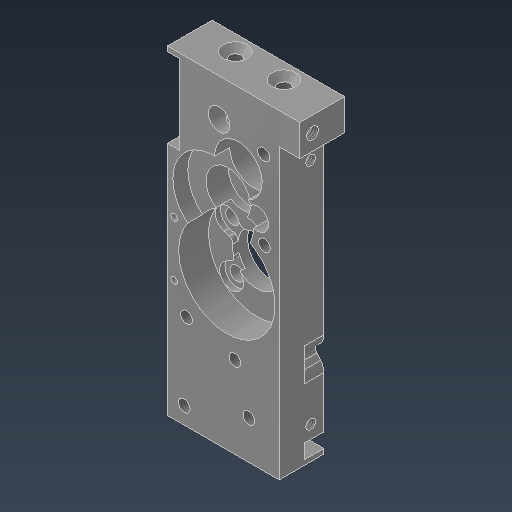
# Autodesk Inventor part: RightGearbox
Saved by Autodesk Inventor 2027.1 (Build 311270010, 270A)
## iProperties
Created: 2026-04-14
Part Number: RightGearbox
Material: Steel
Document SubType Name: Sheet Metal
Designer: szymo
Density: 7.85 g/cm^3
Appearance: Nylon 6(1)
Mass: 69.272 g
Surface Area: 68.2976 cm^2
Volume: 8.82446 cm^3
Sheet Metal Rule: Default
Author: szymo
Autodesk Inventor part; units mm, degrees
(part 1 of 2)
ref_plane "YZ Plane" through (0, 0, 0) normal (1, 0, 0) x (0, 1, 0)
sketch "Sketch1" plane through (0, 0, 0) normal (0, 0, 1) x (1, 0, 0)
  circle A0 centre (14.75, -14.75) radius 4.929289
  circle A1 centre (14.75, -14.75) radius 14.75 construction
  circle A2 centre (14.7, -55.637072) radius 4.955917
  circle A3 centre (14.7, -55.637072) radius 15.294083 construction
  line L0 (23.2, 0) -> (0, 0)
  line L1 (0, 0) -> (0, -66.431155)
  line L2 (0, -66.431155) -> (23.2, -66.431155)
  line L3 (23.2, -66.431155) -> (23.2, 0)
  circle A4 centre (12.35, -35.568116) radius 5
  line L4 (24.683483, -55.062556) -> (28.658141, -52.767786)
  arc A5 (28.658141, -52.767786) -> (24.908656, -45.694948) centre (14.7, -55.637072) ccw
  line L5 (24.908656, -45.694948) -> (21.057709, -47.918294)
  arc A6 (24.683483, -55.062556) -> (21.057709, -47.918294) centre (14.7, -55.637072) ccw construction
  arc A7 (25.213326, -45.342329) -> (3.718756, -65.431155) centre (14.7, -55.637072) ccw
  line L6 (25.213326, -45.342329) -> (3.904013, -59.159587)
  line L7 (6.945596, -62.431155) -> (3.718756, -65.431155)
  line L8 (24.683483, -55.062556) -> (23.2, -55.062556)
  line L9 (24.908656, -45.694948) -> (23.2, -45.694948)
  line L10 (6.945596, -62.431155) -> (3.904013, -59.159587)
  line L11 (24.683483, -55.062556) -> (21.057709, -47.918294)
  line L12 (6.945596, -62.431155) -> (23.2, -62.431155)
  circle A8 centre (9.53986, -23.285481) radius 4.2 construction
  circle A9 centre (9.53986, -23.285481) radius 8 construction
  circle A10 centre (12.35, -35.568116) radius 9.6 construction
  circle A11 centre (12.35, -35.568116) radius 10
  circle A12 centre (9.53986, -23.285481) radius 4.6
  circle A13 centre (9.53986, -23.285481) radius 8.4
  arc A14 (5.920333, -57.852177) -> (6.945596, -62.431155) centre (14.911835, -58.243191) ccw construction
  line L13 (2.5, -1) -> (1.5, -1)
  line L14 (1.5, -1) -> (1.5, -17)
  line L15 (1.5, -17) -> (2.5, -17)
  line L16 (2.5, -17) -> (2.5, -1)
  line L17 (1.5, -1) -> (1, -1)
  line L18 (1, -1) -> (1, -1)
  line L19 (1, -1) -> (0, -1)
  line L20 (2.5, -17) -> (2.5, -17.5)
  line L21 (2.5, -17.5) -> (1, -17.5)
  line L22 (1, -17.5) -> (1, -17.5)
  line L23 (1, -17.5) -> (0, -17.5)
  line L24 (23.2, 0) -> (27.5, 0)
  line L25 (27.5, 0) -> (27.5, -6.5)
  line L26 (27.5, -6.5) -> (23.2, -6.5)
  line L27 (24.939125, -23.498313) -> (20.93749, -21.187968)
  arc A15 (20.93749, -21.187968) -> (23.43749, -16.857841) centre (14.7, -14.7) ccw
  line L28 (23.43749, -16.857841) -> (27.439125, -19.168186)
  arc A16 (24.939125, -23.498313) -> (27.439125, -19.168186) centre (14.7, -14.7) ccw
  circle A17 centre (14.75, -14.75) radius 14.75 construction
  circle A18 centre (14.75, -14.75) radius 14.25 construction
  circle A19 centre (14.7, -14.7) radius 5
  circle A20 centre (14.7, -14.7) radius 14 construction
  circle A21 centre (14.75, -56.178853) radius 14.75 construction
  circle A22 centre (14.75, -56.178853) radius 14.25
  circle A23 centre (14.75, -56.178853) radius 5.5
  arc A24 (4.562446, -32.844788) -> (3.134688, -32.877758) centre (3.986169, -38.820111) ccw
  arc A25 (3.134688, -32.877758) -> (3.006515, -33.363738) centre (12.35, -35.568116) ccw
  arc A26 (3.006515, -33.363738) -> (4.232302, -34.096559) centre (6.677883, -28.614251) ccw
  arc A27 (4.232302, -34.096559) -> (4.166412, -34.523423) centre (12.35, -35.568116) ccw
  arc A28 (4.166412, -34.523423) -> (2.776708, -34.85252) centre (4.845066, -40.487985) ccw
  arc A29 (2.776708, -34.85252) -> (2.752376, -35.354528) centre (12.35, -35.568116) ccw
  arc A30 (2.752376, -35.354528) -> (4.103739, -35.81648) centre (5.356043, -29.945509) ccw
  arc A31 (4.103739, -35.81648) -> (4.128039, -36.247716) centre (12.35, -35.568116) ccw
  arc A32 (4.128039, -36.247716) -> (2.837127, -36.858557) centre (6.031965, -41.940838) ccw
  arc A33 (2.837127, -36.858557) -> (2.9177, -37.354654) centre (12.35, -35.568116) ccw
  arc A34 (2.9177, -37.354654) -> (4.335578, -37.525547) centre (4.339872, -31.522502) ccw
  arc A35 (4.335578, -37.525547) -> (4.449005, -37.942307) centre (12.35, -35.568116) ccw
  arc A36 (4.449005, -37.942307) -> (3.313304, -38.808195) centre (7.494993, -43.115172) ccw
  arc A37 (3.313304, -38.808195) -> (3.495261, -39.276699) centre (12.35, -35.568116) ccw
  arc A38 (3.495261, -39.276699) -> (4.917685, -39.149064) centre (3.673782, -33.276307) ccw
  arc A39 (4.917685, -39.149064) -> (5.115283, -39.533134) centre (12.35, -35.568116) ccw
  arc A40 (5.115283, -39.533134) -> (4.184428, -40.616227) centre (9.170208, -43.959663) ccw
  arc A41 (4.184428, -40.616227) -> (4.459816, -41.036661) centre (12.35, -35.568116) ccw
  arc A42 (4.459816, -41.036661) -> (5.82462, -40.616077) centre (3.386884, -35.130276) ccw
  arc A43 (5.82462, -40.616077) -> (6.097753, -40.950671) centre (12.35, -35.568116) ccw
  arc A44 (6.097753, -40.950671) -> (5.412426, -42.203631) centre (10.984395, -44.437404) ccw
  arc A45 (5.412426, -42.203631) -> (5.76921, -42.557622) centre (12.35, -35.568116) ccw
  arc A46 (5.76921, -42.557622) -> (7.016746, -41.86247) centre (3.491718, -37.00338) ccw
  arc A47 (7.016746, -41.86247) -> (7.353476, -42.132965) centre (12.35, -35.568116) ccw
  arc A48 (7.353476, -42.132965) -> (6.94363, -43.501032) centre (12.858265, -44.527514) ccw
  arc A49 (6.94363, -43.501032) -> (7.366216, -43.773108) centre (12.35, -35.568116) ccw
  arc A50 (7.366216, -43.773108) -> (8.44196, -42.833769) centre (3.983701, -38.813757) ccw
  arc A51 (8.44196, -42.833769) -> (8.827571, -43.028343) centre (12.35, -35.568116) ccw
  arc A52 (8.827571, -43.028343) -> (8.711118, -44.451726) centre (14.709922, -44.226055) ccw
  arc A53 (8.711118, -44.451726) -> (9.181038, -44.629996) centre (12.35, -35.568116) ccw
  arc A54 (9.181038, -44.629996) -> (10.037974, -43.487524) centre (4.841331, -40.482283) ccw
  arc A55 (10.037974, -43.487524) -> (10.455613, -43.597673) centre (12.35, -35.568116) ccw
  arc A56 (10.455613, -43.597673) -> (10.637643, -45.014164) centre (16.458439, -43.546203) ccw
  arc A57 (10.637643, -45.014164) -> (11.134358, -45.090837) centre (12.35, -35.568116) ccw
  arc A58 (11.134358, -45.090837) -> (11.735035, -43.795164) centre (6.027127, -41.936037) ccw
  arc A59 (11.735035, -43.795164) -> (12.166448, -43.816073) centre (12.35, -35.568116) ccw
  arc A60 (12.166448, -43.816073) -> (12.639006, -45.163764) centre (18.027397, -42.51767) ccw
  arc A61 (12.639006, -45.163764) -> (13.140808, -45.135488) centre (12.35, -35.568116) ccw
  arc A62 (13.140808, -45.135488) -> (13.458973, -43.743241) centre (7.489262, -43.111482) ccw
  arc A63 (13.458973, -43.743241) -> (13.885306, -43.673998) centre (12.35, -35.568116) ccw
  arc A64 (13.885306, -43.673998) -> (14.627738, -44.893989) centre (19.348226, -41.185409) ccw
  arc A65 (14.627738, -44.893989) -> (15.112695, -44.762) centre (12.35, -35.568116) ccw
  arc A66 (15.112695, -44.762) -> (15.134444, -43.334027) centre (9.163835, -43.957245) ccw
  arc A67 (15.134444, -43.334027) -> (15.537064, -43.177657) centre (12.35, -35.568116) ccw
  arc A68 (15.537064, -43.177657) -> (16.516922, -44.216627) centre (20.363199, -39.607644) ccw
  arc A69 (16.516922, -44.216627) -> (16.96384, -43.986695) centre (12.35, -35.568116) ccw
  arc A70 (16.96384, -43.986695) -> (16.68822, -42.585404) centre (10.977658, -44.436364) ccw
  arc A71 (16.68822, -42.585404) -> (17.049532, -42.348743) centre (12.35, -35.568116) ccw
  arc A72 (17.049532, -42.348743) -> (18.223992, -43.161285) centre (21.027956, -37.853333) ccw
  arc A73 (18.223992, -43.161285) -> (18.613337, -42.843458) centre (12.35, -35.568116) ccw
  arc A74 (18.613337, -42.843458) -> (18.052396, -41.530093) centre (12.85146, -44.527897) ccw
  arc A75 (18.052396, -41.530093) -> (18.356607, -41.223482) centre (12.35, -35.568116) ccw
  arc A76 (18.356607, -41.223482) -> (19.67434, -41.774084) centre (21.313446, -35.999147) ccw
  arc A77 (19.67434, -41.774084) -> (19.989097, -41.382253) centre (12.35, -35.568116) ccw
  arc A78 (19.989097, -41.382253) -> (19.16735, -40.214215) centre (14.703345, -44.227845) ccw
  arc A79 (19.16735, -40.214215) -> (19.401165, -39.851055) centre (12.35, -35.568116) ccw
  arc A80 (19.401165, -39.851055) -> (20.804579, -40.115653) centre (21.207189, -34.126123) ccw
  arc A81 (20.804579, -40.115653) -> (21.030992, -39.666943) centre (12.35, -35.568116) ccw
  arc A82 (21.030992, -39.666943) -> (19.984353, -38.695279) centre (16.452378, -43.549321) ccw
  arc A83 (19.984353, -38.695279) -> (20.137554, -38.291443) centre (12.35, -35.568116) ccw
  arc A84 (20.137554, -38.291443) -> (21.565312, -38.258473) centre (20.713831, -32.316121) ccw
  arc A85 (21.565312, -38.258473) -> (21.693485, -37.772494) centre (12.35, -35.568116) ccw
  arc A86 (21.693485, -37.772494) -> (20.467698, -37.039672) centre (18.022117, -42.52198) ccw
  arc A87 (20.467698, -37.039672) -> (20.533588, -36.612808) centre (12.35, -35.568116) ccw
  arc A88 (20.533588, -36.612808) -> (21.923292, -36.283711) centre (19.854934, -30.648246) ccw
  arc A89 (21.923292, -36.283711) -> (21.947624, -35.781703) centre (12.35, -35.568116) ccw
  arc A90 (21.947624, -35.781703) -> (20.596261, -35.319751) centre (19.343957, -41.190722) ccw
  arc A91 (20.596261, -35.319751) -> (20.571961, -34.888515) centre (12.35, -35.568116) ccw
  arc A92 (20.571961, -34.888515) -> (21.862873, -34.277674) centre (18.668035, -29.195394) ccw
  arc A93 (21.862873, -34.277674) -> (21.7823, -33.781577) centre (12.35, -35.568116) ccw
  arc A94 (21.7823, -33.781577) -> (20.364422, -33.610684) centre (20.360128, -39.613729) ccw
  arc A95 (20.364422, -33.610684) -> (20.250995, -33.193924) centre (12.35, -35.568116) ccw
  arc A96 (20.250995, -33.193924) -> (21.386696, -32.328036) centre (17.205007, -28.02106) ccw
  arc A97 (21.386696, -32.328036) -> (21.204739, -31.859532) centre (12.35, -35.568116) ccw
  arc A98 (21.204739, -31.859532) -> (19.782315, -31.987167) centre (21.026218, -37.859924) ccw
  arc A99 (19.782315, -31.987167) -> (19.584717, -31.603097) centre (12.35, -35.568116) ccw
  arc A100 (19.584717, -31.603097) -> (20.515572, -30.520004) centre (15.529792, -27.176568) ccw
  arc A101 (20.515572, -30.520004) -> (20.240184, -30.09957) centre (12.35, -35.568116) ccw
  arc A102 (20.240184, -30.09957) -> (18.87538, -30.520154) centre (21.313116, -36.005955) ccw
  arc A103 (18.87538, -30.520154) -> (18.602247, -30.18556) centre (12.35, -35.568116) ccw
  arc A104 (18.602247, -30.18556) -> (19.287574, -28.9326) centre (13.715605, -26.698828) ccw
  arc A105 (19.287574, -28.9326) -> (18.93079, -28.578609) centre (12.35, -35.568116) ccw
  arc A106 (18.93079, -28.578609) -> (17.683254, -29.273761) centre (21.208282, -34.132851) ccw
  arc A107 (17.683254, -29.273761) -> (17.346524, -29.003266) centre (12.35, -35.568116) ccw
  arc A108 (17.346524, -29.003266) -> (17.75637, -27.635199) centre (11.841735, -26.608717) ccw
  arc A109 (17.75637, -27.635199) -> (17.333784, -27.363123) centre (12.35, -35.568116) ccw
  arc A110 (17.333784, -27.363123) -> (16.25804, -28.302462) centre (20.716299, -32.322474) ccw
  arc A111 (16.25804, -28.302462) -> (15.872429, -28.107888) centre (12.35, -35.568116) ccw
  arc A112 (15.872429, -28.107888) -> (15.988882, -26.684505) centre (9.990078, -26.910176) ccw
  arc A113 (15.988882, -26.684505) -> (15.518962, -26.506235) centre (12.35, -35.568116) ccw
  arc A114 (15.518962, -26.506235) -> (14.662026, -27.648707) centre (19.858669, -30.653948) ccw
  arc A115 (14.662026, -27.648707) -> (14.244387, -27.538558) centre (12.35, -35.568116) ccw
  arc A116 (14.244387, -27.538558) -> (14.062357, -26.122067) centre (8.241561, -27.590028) ccw
  arc A117 (14.062357, -26.122067) -> (13.565642, -26.045395) centre (12.35, -35.568116) ccw
  arc A118 (13.565642, -26.045395) -> (12.964965, -27.341068) centre (18.672873, -29.200194) ccw
  arc A119 (12.964965, -27.341068) -> (12.533552, -27.320158) centre (12.35, -35.568116) ccw
  arc A120 (12.533552, -27.320158) -> (12.060994, -25.972467) centre (6.672603, -28.618561) ccw
  arc A121 (12.060994, -25.972467) -> (11.559192, -26.000743) centre (12.35, -35.568116) ccw
  arc A122 (11.559192, -26.000743) -> (11.241027, -27.39299) centre (17.210738, -28.024749) ccw
  arc A123 (11.241027, -27.39299) -> (10.814694, -27.462233) centre (12.35, -35.568116) ccw
  arc A124 (10.814694, -27.462233) -> (10.072262, -26.242243) centre (5.351774, -29.950823) ccw
  arc A125 (10.072262, -26.242243) -> (9.587305, -26.374231) centre (12.35, -35.568116) ccw
  arc A126 (9.587305, -26.374231) -> (9.565556, -27.802205) centre (15.536165, -27.178986) ccw
  arc A127 (9.565556, -27.802205) -> (9.162936, -27.958574) centre (12.35, -35.568116) ccw
  arc A128 (9.162936, -27.958574) -> (8.183078, -26.919604) centre (4.336801, -31.528587) ccw
  arc A129 (8.183078, -26.919604) -> (7.73616, -27.149536) centre (12.35, -35.568116) ccw
  arc A130 (7.73616, -27.149536) -> (8.01178, -28.550827) centre (13.722342, -26.699867) ccw
  arc A131 (8.01178, -28.550827) -> (7.650468, -28.787489) centre (12.35, -35.568116) ccw
  arc A132 (7.650468, -28.787489) -> (6.476008, -27.974946) centre (3.672044, -33.282898) ccw
  arc A133 (6.476008, -27.974946) -> (6.086663, -28.292773) centre (12.35, -35.568116) ccw
  arc A134 (6.086663, -28.292773) -> (6.647604, -29.606138) centre (11.84854, -26.608334) ccw
  arc A135 (6.647604, -29.606138) -> (6.343393, -29.912749) centre (12.35, -35.568116) ccw
  arc A136 (6.343393, -29.912749) -> (5.02566, -29.362147) centre (3.386554, -35.137084) ccw
  arc A137 (5.02566, -29.362147) -> (4.710903, -29.753978) centre (12.35, -35.568116) ccw
  arc A138 (4.710903, -29.753978) -> (5.53265, -30.922016) centre (9.996655, -26.908386) ccw
  arc A139 (5.53265, -30.922016) -> (5.298835, -31.285176) centre (12.35, -35.568116) ccw
  arc A140 (5.298835, -31.285176) -> (3.895421, -31.020578) centre (3.492811, -37.010108) ccw
  arc A141 (3.895421, -31.020578) -> (3.669008, -31.469289) centre (12.35, -35.568116) ccw
  arc A142 (3.669008, -31.469289) -> (4.715647, -32.440952) centre (8.247622, -27.58691) ccw
  arc A143 (4.715647, -32.440952) -> (4.562446, -32.844788) centre (12.35, -35.568116) ccw
  circle A144 centre (9.53986, -23.285481) radius 1.25
  arc A145 (17.496499, -22.453679) -> (16.330814, -22.213772) centre (15.912387, -27.198781) ccw
  arc A146 (16.330814, -22.213772) -> (16.265418, -21.859829) centre (9.53986, -23.285481) ccw
  arc A147 (16.265418, -21.859829) -> (17.268417, -21.219228) centre (14.093328, -17.353454) ccw
  arc A148 (17.268417, -21.219228) -> (17.149686, -20.817578) centre (9.53986, -23.285481) ccw
  arc A149 (17.149686, -20.817578) -> (15.959595, -20.825272) centre (16.586753, -25.788343) ccw
  arc A150 (15.959595, -20.825272) -> (15.822039, -20.492661) centre (9.53986, -23.285481) ccw
  arc A151 (15.822039, -20.492661) -> (16.669931, -19.657523) centre (12.760486, -16.536364) ccw
  arc A152 (16.669931, -19.657523) -> (16.470287, -19.289336) centre (9.53986, -23.285481) ccw
  arc A153 (16.470287, -19.289336) -> (15.307802, -19.544296) centre (16.953135, -24.268518) ccw
  arc A154 (15.307802, -19.544296) -> (15.104099, -19.247552) centre (9.53986, -23.285481) ccw
  arc A155 (15.104099, -19.247552) -> (15.759827, -18.254377) centre (11.286887, -16.014242) ccw
  arc A156 (15.759827, -18.254377) -> (15.487995, -17.935744) centre (9.53986, -23.285481) ccw
  arc A157 (15.487995, -17.935744) -> (14.403922, -18.426827) centre (16.995522, -22.705729) ccw
  arc A158 (14.403922, -18.426827) -> (14.142974, -18.17892) centre (9.53986, -23.285481) ccw
  arc A159 (14.142974, -18.17892) -> (14.577881, -17.071115) centre (9.736935, -15.809909) ccw
  arc A160 (14.577881, -17.071115) -> (14.245741, -16.815962) centre (9.53986, -23.285481) ccw
  arc A161 (14.245741, -16.815962) -> (13.28746, -17.521705) centre (16.712061, -21.168279) ccw
  arc A162 (13.28746, -17.521705) -> (12.980671, -17.33347) centre (9.53986, -23.285481) ccw
  arc A163 (12.980671, -17.33347) -> (13.175748, -16.15945) centre (8.178369, -15.932294) ccw
  arc A164 (13.175748, -16.15945) -> (12.797818, -15.978929) centre (9.53986, -23.285481) ccw
  arc A165 (12.797818, -15.978929) -> (12.007209, -16.868487) centre (16.11514, -19.72336) ccw
  arc A166 (12.007209, -16.868487) -> (11.667988, -16.74815) centre (9.53986, -23.285481) ccw
  arc A167 (11.667988, -16.74815) -> (11.61471, -15.559227) centre (6.679308, -16.376048) ccw
  arc A168 (11.61471, -15.559227) -> (11.207506, -15.461227) centre (9.53986, -23.285481) ccw
  arc A169 (11.207506, -15.461227) -> (10.619124, -16.495723) centre (15.230848, -18.434124) ccw
  arc A170 (10.619124, -16.495723) -> (10.262296, -16.448544) centre (9.53986, -23.285481) ccw
  arc A171 (10.262296, -16.448544) -> (9.962991, -15.296679) centre (5.305266, -17.121778) ccw
  arc A172 (9.962991, -15.296679) -> (9.54431, -15.285482) centre (9.53986, -23.285481) ccw
  arc A173 (9.54431, -15.285482) -> (9.183869, -16.419704) centre (14.097832, -17.356914) ccw
  arc A174 (9.183869, -16.419704) -> (8.82503, -16.447744) centre (9.53986, -23.285481) ccw
  arc A175 (8.82503, -16.447744) -> (8.29278, -15.383279) centre (4.116296, -18.136891) ccw
  arc A176 (8.29278, -15.383279) -> (7.880919, -15.459376) centre (9.53986, -23.285481) ccw
  arc A177 (7.880919, -15.459376) -> (7.764173, -16.643752) centre (12.765611, -16.538812) ccw
  arc A178 (7.764173, -16.643752) -> (7.419005, -16.745787) centre (9.53986, -23.285481) ccw
  arc A179 (7.419005, -16.745787) -> (6.677071, -15.815244) centre (3.164362, -19.377023) ccw
  arc A180 (6.677071, -15.815244) -> (6.290033, -15.975308) centre (9.53986, -23.285481) ccw
  arc A181 (6.290033, -15.975308) -> (6.422083, -17.158076) centre (11.29241, -16.015571) ccw
  arc A182 (6.422083, -17.158076) -> (6.105672, -17.329645) centre (9.53986, -23.285481) ccw
  arc A183 (6.105672, -17.329645) -> (5.18648, -16.573694) centre (2.491067, -20.787972) ccw
  arc A184 (5.18648, -16.573694) -> (4.841179, -16.81073) centre (9.53986, -23.285481) ccw
  arc A185 (4.841179, -16.81073) -> (5.216255, -17.940197) centre (9.742613, -15.810061) ccw
  arc A186 (5.216255, -17.940197) -> (4.94243, -18.173802) centre (9.53986, -23.285481) ccw
  arc A187 (4.94243, -18.173802) -> (3.886153, -17.625481) centre (2.125839, -22.308075) ccw
  arc A188 (3.886153, -17.625481) -> (3.59768, -17.92913) centre (9.53986, -23.285481) ccw
  arc A189 (3.59768, -17.92913) -> (4.199389, -18.955932) centre (8.183955, -15.931262) ccw
  arc A190 (4.199389, -18.955932) -> (3.980117, -19.241364) centre (9.53986, -23.285481) ccw
  arc A191 (3.980117, -19.241364) -> (2.83292, -18.924637) centre (2.084639, -23.870895) ccw
  arc A192 (2.83292, -18.924637) -> (2.613883, -19.281628) centre (9.53986, -23.285481) ccw
  arc A193 (2.613883, -19.281628) -> (3.415927, -20.160889) centre (6.684557, -16.373878) ccw
  arc A194 (3.415927, -20.160889) -> (3.260791, -20.485673) centre (9.53986, -23.285481) ccw
  arc A195 (3.260791, -20.485673) -> (2.072812, -20.414383) centre (2.369268, -25.40813) ccw
  arc A196 (2.072812, -20.414383) -> (1.932784, -20.809113) centre (9.53986, -23.285481) ccw
  arc A197 (1.932784, -20.809113) -> (2.90011, -21.502406) centre (5.309949, -17.118564) ccw
  arc A198 (2.90011, -21.502406) -> (2.815891, -21.852347) centre (9.53986, -23.285481) ccw
  arc A199 (2.815891, -21.852347) -> (1.63905, -22.02961) centre (2.967286, -26.852595) ccw
  arc A200 (1.63905, -22.02961) -> (1.584151, -22.444827) centre (9.53986, -23.285481) ccw
  arc A201 (1.584151, -22.444827) -> (2.674483, -22.921852) centre (4.120208, -18.132773) ccw
  arc A202 (2.674483, -22.921852) -> (2.664861, -23.281657) centre (9.53986, -23.285481) ccw
  arc A203 (2.664861, -23.281657) -> (1.550592, -23.699724) centre (3.852558, -28.14116) ccw
  arc A204 (1.550592, -23.699724) -> (1.58322, -24.117283) centre (9.53986, -23.285481) ccw
  arc A205 (1.58322, -24.117283) -> (2.748905, -24.35719) centre (3.167332, -19.372181) ccw
  arc A206 (2.748905, -24.35719) -> (2.814301, -24.711133) centre (9.53986, -23.285481) ccw
  arc A207 (2.814301, -24.711133) -> (1.811302, -25.351734) centre (4.986391, -29.217508) ccw
  arc A208 (1.811302, -25.351734) -> (1.930033, -25.753384) centre (9.53986, -23.285481) ccw
  arc A209 (1.930033, -25.753384) -> (3.120125, -25.74569) centre (2.492967, -20.782619) ccw
  arc A210 (3.120125, -25.74569) -> (3.25768, -26.078301) centre (9.53986, -23.285481) ccw
  arc A211 (3.25768, -26.078301) -> (2.409788, -26.913439) centre (6.319233, -30.034598) ccw
  arc A212 (2.409788, -26.913439) -> (2.609432, -27.281626) centre (9.53986, -23.285481) ccw
  arc A213 (2.609432, -27.281626) -> (3.771917, -27.026666) centre (2.126584, -22.302444) ccw
  arc A214 (3.771917, -27.026666) -> (3.975621, -27.32341) centre (9.53986, -23.285481) ccw
  arc A215 (3.975621, -27.32341) -> (3.319892, -28.316585) centre (7.792832, -30.55672) ccw
  arc A216 (3.319892, -28.316585) -> (3.591724, -28.635218) centre (9.53986, -23.285481) ccw
  arc A217 (3.591724, -28.635218) -> (4.675797, -28.144135) centre (2.084197, -23.865233) ccw
  arc A218 (4.675797, -28.144135) -> (4.936745, -28.392042) centre (9.53986, -23.285481) ccw
  arc A219 (4.936745, -28.392042) -> (4.501839, -29.499847) centre (9.342784, -30.761053) ccw
  arc A220 (4.501839, -29.499847) -> (4.833978, -29.755) centre (9.53986, -23.285481) ccw
  arc A221 (4.833978, -29.755) -> (5.792259, -29.049257) centre (2.367658, -25.402683) ccw
  arc A222 (5.792259, -29.049257) -> (6.099048, -29.237493) centre (9.53986, -23.285481) ccw
  arc A223 (6.099048, -29.237493) -> (5.903971, -30.411512) centre (10.90135, -30.638668) ccw
  arc A224 (5.903971, -30.411512) -> (6.281901, -30.592033) centre (9.53986, -23.285481) ccw
  arc A225 (6.281901, -30.592033) -> (7.07251, -29.702475) centre (2.964579, -26.847602) ccw
  arc A226 (7.07251, -29.702475) -> (7.411731, -29.822812) centre (9.53986, -23.285481) ccw
  arc A227 (7.411731, -29.822812) -> (7.465009, -31.011735) centre (12.400412, -30.194914) ccw
  arc A228 (7.465009, -31.011735) -> (7.872213, -31.109735) centre (9.53986, -23.285481) ccw
  arc A229 (7.872213, -31.109735) -> (8.460595, -30.075239) centre (3.848871, -28.136839) ccw
  arc A230 (8.460595, -30.075239) -> (8.817423, -30.122418) centre (9.53986, -23.285481) ccw
  arc A231 (8.817423, -30.122418) -> (9.116728, -31.274283) centre (13.774453, -29.449184) ccw
  arc A232 (9.116728, -31.274283) -> (9.535409, -31.28548) centre (9.53986, -23.285481) ccw
  arc A233 (9.535409, -31.28548) -> (9.89585, -30.151258) centre (4.981887, -29.214048) ccw
  arc A234 (9.89585, -30.151258) -> (10.254689, -30.123218) centre (9.53986, -23.285481) ccw
  arc A235 (10.254689, -30.123218) -> (10.78694, -31.187683) centre (14.963423, -28.434071) ccw
  arc A236 (10.78694, -31.187683) -> (11.1988, -31.111586) centre (9.53986, -23.285481) ccw
  arc A237 (11.1988, -31.111586) -> (11.315546, -29.92721) centre (6.314108, -30.03215) ccw
  arc A238 (11.315546, -29.92721) -> (11.660714, -29.825175) centre (9.53986, -23.285481) ccw
  arc A239 (11.660714, -29.825175) -> (12.402648, -30.755718) centre (15.915357, -27.193939) ccw
  arc A240 (12.402648, -30.755718) -> (12.789687, -30.595654) centre (9.53986, -23.285481) ccw
  arc A241 (12.789687, -30.595654) -> (12.657636, -29.412886) centre (7.78731, -30.555391) ccw
  arc A242 (12.657636, -29.412886) -> (12.974047, -29.241317) centre (9.53986, -23.285481) ccw
  arc A243 (12.974047, -29.241317) -> (13.893239, -29.997268) centre (16.588652, -25.78299) ccw
  arc A244 (13.893239, -29.997268) -> (14.23854, -29.760232) centre (9.53986, -23.285481) ccw
  arc A245 (14.23854, -29.760232) -> (13.863464, -28.630766) centre (9.337106, -30.760901) ccw
  arc A246 (13.863464, -28.630766) -> (14.13729, -28.39716) centre (9.53986, -23.285481) ccw
  arc A247 (14.13729, -28.39716) -> (15.193566, -28.945481) centre (16.95388, -24.262887) ccw
  arc A248 (15.193566, -28.945481) -> (15.482039, -28.641832) centre (9.53986, -23.285481) ccw
  arc A249 (15.482039, -28.641832) -> (14.88033, -27.61503) centre (10.895764, -30.6397) ccw
  arc A250 (14.88033, -27.61503) -> (15.099603, -27.329598) centre (9.53986, -23.285481) ccw
  arc A251 (15.099603, -27.329598) -> (16.246799, -27.646325) centre (16.99508, -22.700067) ccw
  arc A252 (16.246799, -27.646325) -> (16.465837, -27.289335) centre (9.53986, -23.285481) ccw
  arc A253 (16.465837, -27.289335) -> (15.663792, -26.410073) centre (12.395163, -30.197085) ccw
  arc A254 (15.663792, -26.410073) -> (15.818928, -26.085289) centre (9.53986, -23.285481) ccw
  arc A255 (15.818928, -26.085289) -> (17.006907, -26.156579) centre (16.710451, -21.162832) ccw
  arc A256 (17.006907, -26.156579) -> (17.146935, -25.761849) centre (9.53986, -23.285481) ccw
  arc A257 (17.146935, -25.761849) -> (16.179609, -25.068556) centre (13.769771, -29.452399) ccw
  arc A258 (16.179609, -25.068556) -> (16.263828, -24.718615) centre (9.53986, -23.285481) ccw
  arc A259 (16.263828, -24.718615) -> (17.440669, -24.541352) centre (16.112433, -19.718367) ccw
  arc A260 (17.440669, -24.541352) -> (17.495568, -24.126135) centre (9.53986, -23.285481) ccw
  arc A261 (17.495568, -24.126135) -> (16.405236, -23.64911) centre (14.959511, -28.438189) ccw
  arc A262 (16.405236, -23.64911) -> (16.414859, -23.289306) centre (9.53986, -23.285481) ccw
  arc A263 (16.414859, -23.289306) -> (17.529128, -22.871238) centre (15.227161, -18.429802) ccw
  arc A264 (17.529128, -22.871238) -> (17.496499, -22.453679) centre (9.53986, -23.285481) ccw
  circle A265 centre (9.53986, -23.285481) radius 1.25
  arc A266 (5.771961, -25.140998) -> (7.169291, -24.867538) centre (5.772396, -21.436445) ccw
  arc A267 (7.169291, -24.867538) -> (7.396071, -25.163424) centre (9.53986, -23.285481) ccw
  arc A268 (7.396071, -25.163424) -> (6.768851, -26.441667) centre (10.346218, -27.404037) ccw
  arc A269 (6.768851, -26.441667) -> (7.204522, -26.776355) centre (9.53986, -23.285481) ccw
  arc A270 (7.204522, -26.776355) -> (8.277915, -25.840867) centre (5.352623, -23.567901) ccw
  arc A271 (8.277915, -25.840867) -> (8.622256, -25.983722) centre (9.53986, -23.285481) ccw
  arc A272 (8.622256, -25.983722) -> (8.718189, -27.404323) centre (12.297464, -26.449075) ccw
  arc A273 (8.718189, -27.404323) -> (9.262835, -27.476335) centre (9.53986, -23.285481) ccw
  arc A274 (9.262835, -27.476335) -> (9.724676, -26.129482) centre (6.054816, -25.623682) ccw
  arc A275 (9.724676, -26.129482) -> (10.094312, -26.081028) centre (9.53986, -23.285481) ccw
  arc A276 (10.094312, -26.081028) -> (10.887693, -27.263338) centre (13.509813, -24.646432) ccw
  arc A277 (10.887693, -27.263338) -> (11.395376, -27.053379) centre (9.53986, -23.285481) ccw
  arc A278 (11.395376, -27.053379) -> (11.121916, -25.65605) centre (7.690824, -27.052944) ccw
  arc A279 (11.121916, -25.65605) -> (11.417803, -25.42927) centre (9.53986, -23.285481) ccw
  arc A280 (11.417803, -25.42927) -> (12.696046, -26.05649) centre (13.658415, -22.479122) ccw
  arc A281 (12.696046, -26.05649) -> (13.030733, -25.620818) centre (9.53986, -23.285481) ccw
  arc A282 (13.030733, -25.620818) -> (12.095245, -24.547426) centre (9.822279, -27.472718) ccw
  arc A283 (12.095245, -24.547426) -> (12.2381, -24.203085) centre (9.53986, -23.285481) ccw
  arc A284 (12.2381, -24.203085) -> (13.658701, -24.107152) centre (12.703454, -20.527876) ccw
  arc A285 (13.658701, -24.107152) -> (13.730714, -23.562506) centre (9.53986, -23.285481) ccw
  arc A286 (13.730714, -23.562506) -> (12.383861, -23.100664) centre (11.878061, -26.770525) ccw
  arc A287 (12.383861, -23.100664) -> (12.335406, -22.731029) centre (9.53986, -23.285481) ccw
  arc A288 (12.335406, -22.731029) -> (13.517717, -21.937648) centre (10.90081, -19.315528) ccw
  arc A289 (13.517717, -21.937648) -> (13.307758, -21.429964) centre (9.53986, -23.285481) ccw
  arc A290 (13.307758, -21.429964) -> (11.910428, -21.703424) centre (13.307323, -25.134517) ccw
  arc A291 (11.910428, -21.703424) -> (11.683648, -21.407538) centre (9.53986, -23.285481) ccw
  arc A292 (11.683648, -21.407538) -> (12.310868, -20.129295) centre (8.733501, -19.166926) ccw
  arc A293 (12.310868, -20.129295) -> (11.875197, -19.794607) centre (9.53986, -23.285481) ccw
  arc A294 (11.875197, -19.794607) -> (10.801804, -20.730095) centre (13.727096, -23.003062) ccw
  arc A295 (10.801804, -20.730095) -> (10.457463, -20.58724) centre (9.53986, -23.285481) ccw
  arc A296 (10.457463, -20.58724) -> (10.36153, -19.166639) centre (6.782255, -20.121887) ccw
  arc A297 (10.36153, -19.166639) -> (9.816884, -19.094627) centre (9.53986, -23.285481) ccw
  arc A298 (9.816884, -19.094627) -> (9.355043, -20.44148) centre (13.024903, -20.94728) ccw
  arc A299 (9.355043, -20.44148) -> (8.985407, -20.489934) centre (9.53986, -23.285481) ccw
  arc A300 (8.985407, -20.489934) -> (8.192026, -19.307624) centre (5.569907, -21.92453) ccw
  arc A301 (8.192026, -19.307624) -> (7.684343, -19.517583) centre (9.53986, -23.285481) ccw
  arc A302 (7.684343, -19.517583) -> (7.957803, -20.914912) centre (11.388896, -19.518018) ccw
  arc A303 (7.957803, -20.914912) -> (7.661916, -21.141693) centre (9.53986, -23.285481) ccw
  arc A304 (7.661916, -21.141693) -> (6.383673, -20.514472) centre (5.421304, -24.09184) ccw
  arc A305 (6.383673, -20.514472) -> (6.048986, -20.950144) centre (9.53986, -23.285481) ccw
  arc A306 (6.048986, -20.950144) -> (6.984474, -22.023537) centre (9.25744, -19.098244) ccw
  arc A307 (6.984474, -22.023537) -> (6.841619, -22.367877) centre (9.53986, -23.285481) ccw
  arc A308 (6.841619, -22.367877) -> (5.421018, -22.46381) centre (6.376265, -26.043086) ccw
  arc A309 (5.421018, -22.46381) -> (5.349006, -23.008457) centre (9.53986, -23.285481) ccw
  arc A310 (5.349006, -23.008457) -> (6.695858, -23.470298) centre (7.201659, -19.800437) ccw
  arc A311 (6.695858, -23.470298) -> (6.744313, -23.839933) centre (9.53986, -23.285481) ccw
  arc A312 (6.744313, -23.839933) -> (5.562003, -24.633314) centre (8.178909, -27.255434) ccw
  arc A313 (5.562003, -24.633314) -> (5.771961, -25.140998) centre (9.53986, -23.285481) ccw
  line L29 (1.5, -17) -> (1.5, -1)
  line L30 (2.5, -17) -> (1.5, -17)
  line L31 (2.5, -1) -> (2.5, -17)
  line L32 (2.5, -1) -> (1.5, -1)
  line L33 (3.718756, -65.431155) -> (23.2, -65.431155)
  line L34 (1.573155, -59.167706) -> (3.584849, -58.006254)
  arc A314 (5.054408, -58.627423) -> (3.584849, -58.006254) centre (4.084849, -58.872279) ccw
  arc A315 (5.054408, -58.627423) -> (7.781681, -63.351197) centre (14.75, -56.178853) ccw
  arc A316 (7.584849, -64.934457) -> (7.781681, -63.351197) centre (7.084849, -64.068432) ccw
  line L35 (7.584849, -64.934457) -> (5.573155, -66.095909)
  arc A317 (4.342827, -65.912981) -> (5.573155, -66.095909) centre (5.073155, -65.229884) ccw
  arc A318 (4.342827, -65.912981) -> (28.383589, -52.03304) centre (14.75, -56.178853) ccw
  arc A319 (27.926845, -53.19) -> (28.383589, -52.03304) centre (27.426845, -52.323975) ccw
  line L36 (27.926845, -53.19) -> (25.915151, -54.351452)
  arc A320 (24.445592, -53.730284) -> (25.915151, -54.351452) centre (25.415151, -53.485427) ccw
  arc A321 (24.445592, -53.730284) -> (21.718319, -49.006509) centre (14.75, -56.178853) ccw
  arc A322 (21.915151, -47.423249) -> (21.718319, -49.006509) centre (22.415151, -48.289274) ccw
  line L37 (21.915151, -47.423249) -> (23.926845, -46.261797)
  arc A323 (25.157173, -46.444725) -> (23.926845, -46.261797) centre (24.426845, -47.127822) ccw
  arc A324 (25.157173, -46.444725) -> (1.116411, -60.324666) centre (14.75, -56.178853) ccw
  arc A325 (1.573155, -59.167706) -> (1.116411, -60.324666) centre (2.073155, -60.033732) ccw
  arc A326 (2.65398, -7.21682) -> (2.795717, -8.452571) centre (3.502824, -7.745464) ccw
  arc A327 (7.21682, -2.65398) -> (2.65398, -7.21682) centre (14.75, -14.75) ccw
  arc A328 (8.452571, -2.795717) -> (7.21682, -2.65398) centre (7.745464, -3.502824) ccw
  line L38 (10.095112, -4.438258) -> (8.452571, -2.795717)
  arc A329 (9.87546, -6.018514) -> (10.095112, -4.438258) centre (9.388006, -5.145365) ccw
  arc A330 (9.87546, -6.018514) -> (6.018514, -9.87546) centre (14.75, -14.75) ccw
  arc A331 (4.438258, -10.095112) -> (6.018514, -9.87546) centre (5.145365, -9.388006) ccw
  line L39 (2.795717, -8.452571) -> (4.438258, -10.095112)
  point P0 (0, 0)
  point P1 (4.394176, -65.837072)
  point P2 (4.201679, -29.771145)
  point P3 (9.822706, -14.890244)
  point P4 (16.877474, -19.196543)
  point P5 (17.167076, -26.804795)
  point P6 (6.999126, -27.120148)
  point P7 (13.495221, -25.633909)
  point P8 (10.057406, -65.837072)
  point P9 (22.512272, -49.394604)
  point P10 (24.012272, -51.99268)
  point P11 (5.387728, -59.281464)
  point P12 (6.887728, -61.87954)
  point P13 (23.2, -46.681441)
  point P14 (23.2, -52.139486)
  point P15 (0, -56.286515)
  point P16 (0, -54.98763)
  point P17 (24.401437, -45.694948)
  point P18 (24.511534, -45.797381)
  point P19 (24.669508, -45.694948)
  point P20 (16.527844, -50.974118)
  point P21 (14.244563, -50.702127)
  point P22 (16.473504, -51.009352)
  point P23 (1.116411, -60.324666)
  point P24 (4.342827, -65.912981)
  point P25 (6.724542, -65.431155)
  point P26 (21.915151, -47.423249)
  point P27 (23.2, -50.83119)
  dimension "d2" = 4.5
  dimension "d3" = 6.3
  dimension "d4" = 0.4
  dimension "d5" = 0.4
  dimension "d6" = 0.4
  dimension "d27" = 0
  dimension "d36" = 0.5
  dimension "d37" = 0
  dimension "d38" = 0.5
  dimension "d39" = 0.5
  dimension "d40" = 0
  dimension "d41" = 2
  dimension "d43" = 10
  dimension "d112" = 6.5
  dimension "d231" = 1
  dimension "d232" = 3
  constraints: 60 end point, 14 centre point, 13 perpendicular, 12 point on circle, 10 coincident, 7 point on line, 6 tangent, 5 parallel, 4 horizontal, 3 collinear, 1 equal radius, 1 vertical, 17 other
  measures "d2" distance edge to line of A3 L2
  measures "d3" distance edge to line of A1 L3
  measures "d27" distance from line of L6 A14.start
  measures "d36" distance between parallel lines of L14 L18
  measures "d37" distance between parallel lines of L19 L13
  measures "d38" distance between parallel lines of L22 L14
  measures "d39" distance between parallel lines of L21 L15
  measures "d40" distance between parallel lines of L21 L23
  measures "d41" distance edge to line of A1 L25
  measures "d43" diameter of A4
  measures "d112" distance between parallel lines of L26 L24
  measures "d231" distance between parallel lines of L2 L33
  measures "d232" distance between parallel lines of L33 L12
extrude "Extrusion5" add sketch "Sketch1" along normal blind 3.1 contours A0 A13 A19 | A0 A172 A19 A13 | A19 A13 A11 A7 L1 L23 L21 L20 L16 L13 L17 L19 L0 L3 A15 L27 | A0 A152 A19 A172 | A13 A19 A152 A0 | A19 A172 A173 A174 A175 A176 A177 A178 A179 A180 A181 A182 A183 A184 A185 A186 A187 A188 A189 A190 A191 A192 A193 A194 A195 A196 A197 A198 A199 A200 A201 A202 A203 A204 A205 A206 A207 A208 A209 A210 A211 A212 A213 A214 A215 A216 A217 A218 A219 A11 A13 | A13 A11 A254 A255 A256 A257 A258 A259 A260 A261 A262 A263 A264 A145 A146 A147 A148 A149 A150 A151 A152 A19 | A19 A152 A151 A150 A149 A148 A147 A146 A145 A264 A263 A262 A261 A260 A259 A258 A257 A256 A255 A254 A11 A12 A219 A218 A217 A216 A215 A214 A213 A212 A211 A210 A209 A208 A207 A206 A205 A204 A203 A202 A201 A200 A199 A198 A197 A196 A195 A194 A193 A192 A191 A190 A189 A188 A187 A186 A185 A184 A183 A182 A181 A180 A179 A178 A177 A176 A175 A174 A173 A172 | A13 A138 A139 A140 A141 A142 A143 A24 A25 A26 A27 A28 A29 A30 A31 A32 A33 A34 A35 A36 A37 A38 A39 A40 A41 A42 A43 A44 A45 A46 A47 A48 A7 A11 | A11 A219 A220 A137 A138 A13 | A11 A12 A130 A131 A132 A133 A134 A135 A136 A223 A222 A221 A137 A220 A219 | A11 A22 L7 A7 L1 | A7 A48 A49 A50 A51 A52 A22 A11 | A138 A137 A220 A221 A136 A223 A224 A225 A226 A227 A228 A229 A230 A231 A232 A233 A234 A235 A4 A13 | A13 A4 A110 A109 A108 A107 A106 A105 A104 A103 A102 A101 A100 A99 A98 A97 A96 A95 A94 A93 A92 A91 A90 A89 A88 A87 A86 A85 A84 A83 A82 A81 A80 A79 A78 A77 A76 A75 A7 A48 A47 A46 A45 A44 A43 A42 A41 A40 A39 A38 A37 A36 A35 A34 A33 A32 A31 A30 A29 A28 A27 A26 A25 A24 A143 A142 A141 A140 A139 A138 | A13 A110 A111 A112 A251 A252 A253 A113 A254 A11 | A11 A7 A75 A76 A77 A78 A79 A80 A81 A82 A83 A84 A85 A86 A87 A88 A89 A90 A91 A92 A93 A94 A95 A96 A97 A98 A99 A100 A101 A102 A103 A104 A105 A106 A107 A108 A109 A110 A13 | A7 A75 A74 A22 A52 A51 A50 A49 A48 | A22 A52 A53 A54 A55 A56 A57 A58 A59 A60 A61 A62 A63 A64 A65 A66 A67 A68 A69 A70 A71 A72 A73 A74 A11 | A11 A22 L3 L6 L5 L11 A23 A314 L34 A325 | A254 A253 A113 A114 A115 A116 A117 A118 A119 A120 A12 A11 | A13 A4 A241 A242 A243 A244 A245 A246 A247 A248 A249 A250 A251 A112 A111 A110 | A12 A128 A127 A120 A119 A118 A117 A116 A115 A114 A113 A253 A112 A251 A250 A249 A248 A247 A246 A245 A244 A243 A242 A241 A4 A239 A238 A237 A235 A234 A233 A232 A231 A230 A229 A228 A227 A226 A225 A224 A223 A136 A135 A134 A133 A132 A131 A130 | A137 A136 A221 A220 | A7 A11 A22 A74 A75 | A7 L33 A22 L2 L1 | A11 A7 L3 A22 | A22 A74 A73 A72 A71 A70 A69 A68 A67 A66 A65 A64 A63 A62 A61 A60 A59 A58 A57 A56 A55 A54 A53 A52 | A325 L34 A314 L6 L10 L7 A22 | A12 A127 A128 | L7 A22 L33 | L7 A315 A316 L35 L33 A22 | A237 A238 A239 A4 | A113 A112 A253 | A221 A222 A223 A136 | A22 A317 L35 L33 L3 L2 | L33 L35 A317 A22 | A315 A314 L6 A23 L11 L3 L12 | L10 L6 A314 A315 | L12 L3 L33 L35 A316 A315 | L27 A15 L3 | A253 A252 A251 A112 | L24 L25 L26 L3 | L3 L5 L6 | L3 A321 A322 L6 L5 | L6 A322 L5 | A23 A2 L6 | L6 A2 A23 | L3 L11 L6 A322 A321 | A322 L6 L11 L5 | L6 A2 | A2 L6 | A23 L6 A2 | A327 A328 L38 A329 A330 A331 L39 A326 picked at (11.538074, -10.990692)
extrude "Extrusion6" add sketch "Sketch1" along normal blind 6.2 contours A0 A13 A19 | A0 A172 A19 A13 | A19 A13 A11 A7 L1 L23 L21 L20 L16 L13 L17 L19 L0 L3 A15 L27 | A0 A152 A19 A172 | A13 A19 A152 A0 | A19 A172 A173 A174 A175 A176 A177 A178 A179 A180 A181 A182 A183 A184 A185 A186 A187 A188 A189 A190 A191 A192 A193 A194 A195 A196 A197 A198 A199 A200 A201 A202 A203 A204 A205 A206 A207 A208 A209 A210 A211 A212 A213 A214 A215 A216 A217 A218 A219 A11 A13 | A13 A11 A254 A255 A256 A257 A258 A259 A260 A261 A262 A263 A264 A145 A146 A147 A148 A149 A150 A151 A152 A19 | A19 A152 A151 A150 A149 A148 A147 A146 A145 A264 A263 A262 A261 A260 A259 A258 A257 A256 A255 A254 A11 A12 A219 A218 A217 A216 A215 A214 A213 A212 A211 A210 A209 A208 A207 A206 A205 A204 A203 A202 A201 A200 A199 A198 A197 A196 A195 A194 A193 A192 A191 A190 A189 A188 A187 A186 A185 A184 A183 A182 A181 A180 A179 A178 A177 A176 A175 A174 A173 A172 | A11 A22 L7 A7 L1 | A11 A22 L3 L6 L5 L11 A23 A314 L34 A325 | A7 L33 A22 L2 L1 | A11 A7 L3 A22 | A325 L34 A314 L6 L10 L7 A22 | L7 A22 L33 | L7 A315 A316 L35 L33 A22 | A22 A317 L35 L33 L3 L2 | L33 L35 A317 A22 | A315 A314 L6 A23 L11 L3 L12 | L10 L6 A314 A315 | L12 L3 L33 L35 A316 A315 | L27 A15 L3 | L24 L25 L26 L3 | L3 L5 L6 | L3 A321 A322 L6 L5 | L6 A322 L5 | A23 A2 L6 | L6 A2 A23 | L3 L11 L6 A322 A321 | A322 L6 L11 L5 | L6 A2 | A2 L6 | A23 L6 A2 | A327 A328 L38 A329 A330 A331 L39 A326 picked at (11.538074, -10.990692)
ref_plane "Work Plane3" through (6.764102, -40.858111, 9.3) normal (0, 0, 1) x (0.9993859, -0.0350396, 0)
extrude "Extrusion7" add sketch "Sketch1" along normal up to surface (9.3 mm away) contours A0 A13 A19 | A19 A13 A11 A7 L1 L23 L21 L20 L16 L13 L17 L19 L0 L3 A15 L27 | A11 A22 L7 A7 L1 | A11 A22 L3 L6 L5 L11 A23 A314 L34 A325 | A7 L33 A22 L2 L1 | A11 A7 L3 A22 | A325 L34 A314 L6 L10 L7 A22 | L7 A22 L33 | L7 A315 A316 L35 L33 A22 | A22 A317 L35 L33 L3 L2 | L33 L35 A317 A22 | A315 A314 L6 A23 L11 L3 L12 | L10 L6 A314 A315 | L12 L3 L33 L35 A316 A315 | L27 A15 L3 | L24 L25 L26 L3 | L3 L5 L6 | L3 A321 A322 L6 L5 | L6 A322 L5 | A23 A2 L6 | L6 A2 A23 | L3 L11 L6 A322 A321 | A322 L6 L11 L5 | L6 A2 | A2 L6 | A23 L6 A2 | A327 A328 L38 A329 A330 A331 L39 A326 picked at (11.538074, -10.990692)
extrude "Extrusion8" cut sketch "Sketch1" along normal blind 4 contours L1 A7 | A325 L34 A314 L6 L10 L7 A22 | L7 A315 A316 L35 L33 A22 | L33 L35 A317 A22 | L9 L6 A22 | L10 L6 A314 A315 | L12 L3 L33 L35 A316 A315 | L3 A321 A322 L6 L5 | L6 A322 L5 | A23 A2 L6 | L6 A2 A23 | L6 A2 | A2 L6 | A23 L6 A2
sketch "Sketch3" plane through (0, -66.431155, 9.3) normal (0, -1, 0) x (1, 0, 0)
  line L0 (23.2, -9.3) -> (23.2, 0) projected
  line L1 (23.2, 0) -> (0, 0) projected
  line L2 (0, -9.3) -> (0, 0) projected
  circle A0 centre (13.6, -3) radius 3
  circle A1 centre (7, -3) radius 3
  line L3 (4, -9.3) -> (4, 0)
  line L4 (0, -9.3) -> (23.2, -9.3) projected
  circle A2 centre (20.2, -3) radius 3
  line L5 (23.2, -9.3) -> (23.2, 0) projected
  line L6 (23.2, 0) -> (0, 0) projected
  point P0 (0, -9.3)
  dimension "d71" = 6
  dimension "d72" = 6
  dimension "d73" = 4
  dimension "d188" = 6
  dimension "d189" = 6.6
  dimension "d190" = 6.6
  constraints: 5 tangent, 3 centre point, 2 end point, 1 perpendicular, 1 point on line
  measures "d71" diameter of A1
  measures "d72" diameter of A0
  measures "d73" distance between parallel lines of L2 L3
  measures "d188" diameter of A2
  measures "d189" distance of A0.centre A2.centre
  measures "d190" distance of A1.centre A0.centre
hole "Hole1" at (13.6, -66.431155, 6.3) at (7, -66.431155, 6.3) at (20.2, -66.431155, 6.3) direction (0, 1, 0) diameter 2.459 depth 10 thread size "M3x0.5" class "6H" standard "ISO Metric profile"
sketch "Sketch4" plane through (0, 0, 9.3) normal (0, 0, 1) x (1, 0, 0)
  arc A0 (4.201679, -29.771145) -> (17.167076, -26.804795) centre (12.35, -35.568116) ccw
  arc A1 (9.822706, -14.890244) -> (4.201679, -29.771145) centre (9.53986, -23.285481) ccw
  arc A2 (16.877474, -19.196543) -> (9.822706, -14.890244) centre (14.75, -14.75) ccw
  arc A3 (17.167076, -26.804795) -> (16.877474, -19.196543) centre (9.53986, -23.285481) ccw
  line L0 (27.5, 0) -> (27.5, -6.5)
  line L1 (0, 0) -> (27.5, 0)
  line L2 (0, -1) -> (0, 0)
  line L3 (2.5, -1) -> (0, -1)
  line L4 (2.5, -17.5) -> (2.5, -1)
  line L5 (0, -17.5) -> (2.5, -17.5)
  line L6 (0, -66.431155) -> (0, -17.5)
  line L7 (23.2, -6.5) -> (23.2, -66.431155)
  line L8 (27.5, -6.5) -> (23.2, -6.5)
  line L9 (23.2, -6.5) -> (2.5, -6.5)
  line L10 (23.2, -19.5) -> (2.5, -19.5)
  circle A4 centre (16.9, -58.431155) radius 3
  circle A5 centre (3.5, -62.931155) radius 3.5
  line L11 (0, -66.431155) -> (0, 0)
  line L12 (23.2, -66.431155) -> (0, -66.431155)
  line L13 (23.2, -6.5) -> (23.2, -66.431155)
  circle A6 centre (20.0066, -9.5) radius 3
  circle A7 centre (20.0066, -9.5) radius 2.5
  arc A8 (16.877474, -19.196543) -> (9.822706, -14.890244) centre (14.75, -14.75) ccw
  circle A9 centre (4, -46.805442) radius 4
  circle A10 centre (14, -49.470543) radius 4
  arc A11 (4.201679, -29.771145) -> (17.167076, -26.804795) centre (12.35, -35.568116) ccw
  circle A12 centre (20.146454, -25.797481) radius 3
  circle A13 centre (20.146454, -25.797481) radius 2.5
  line L14 (23.2, -66.431155) -> (0, -66.431155)
  line L15 (21.4295, -66.431155) -> (18.9705, -66.431155)
  line L16 (14.8295, -66.431155) -> (12.3705, -66.431155)
  line L17 (12.3705, -56.431155) -> (14.8295, -56.431155)
  line L18 (21.4295, -66.431155) -> (18.9705, -66.431155)
  line L19 (18.9705, -56.431155) -> (21.4295, -56.431155)
  point P0 (0, -15)
  dimension "d85" = 6.5
  dimension "d86" = 19.5
  dimension "d87" = 6
  dimension "d88" = 7
  dimension "d89" = 6
  dimension "d90" = 5
  dimension "d92" = 8
  dimension "d93" = 8
  dimension "d94" = 6
  dimension "d95" = 5
  dimension "d103" = 10
  dimension "d191" = 5
  dimension "d192" = 4.5295
  dimension "d193" = 4.5295
  constraints: 9 tangent, 8 centre point, 4 end point, 4 point on line, 2 coincident, 1 parallel, 1 perpendicular
  measures "d85" distance between parallel lines of L1 L9
  measures "d86" distance between parallel lines of L1 L10
  measures "d87" diameter of A4
  measures "d88" diameter of A5
  measures "d89" diameter of A6
  measures "d90" diameter of A7
  measures "d92" diameter of A9
  measures "d93" diameter of A10
  measures "d94" diameter of A12
  measures "d95" diameter of A13
  measures "d103" horizontal distance of A9.centre A10.centre
  measures "d191" distance edge to line of A4 L12
  measures "d192" horizontal distance of A4.centre L19.end
  measures "d193" horizontal distance of A4.centre L17.start
sketch "Sketch12" plane through (0, 0, 9.3) normal (0, 0, 1) x (1, 0, 0)
  circle A0 centre (18.75, -21.678203) radius 1.05643
  circle A1 centre (10.75, -7.821797) radius 1.05643
  circle A2 centre (14.75, -14.75) radius 5.5
  circle A3 centre (14.75, -14.75) radius 14.25
  point P0 (0, 0)
hole "Hole9" at (10.75, -7.821797, 9.3) at (18.75, -21.678203, 9.3) direction (0, 0, -1) diameter 2.5 depth 10.3 counterbore diameter 4.5 counterbore depth 5.3
hole "Hole2" at (14, -49.470543, 9.3) at (20.146454, -25.797481, 9.3) at (16.9, -58.431155, 9.3) at (3.5, -62.931155, 9.3) at (4, -46.805442, 9.3) at (20.0066, -9.5, 9.3) direction (0, 0, -1) diameter 2.459 depth 15.55 thread size "M3x0.5" class "6H" standard "ISO Metric profile"
sketch "Sketch6" plane through (27.5, -6.5, 0) normal (1, 0, 0) x (0, 0, -1)
  line L0 (0, 0) -> (0, 6.5) projected
  line L1 (0, 6.5) -> (-9.3, 6.5) projected
  line L2 (-9.3, 6.5) -> (-9.3, 0) projected
  line L3 (0, 0) -> (-9.3, 0) projected
  line L4 (-4, 0) -> (-4, 6.5)
  line L5 (0, 0) -> (-9.3, 0) projected
  line L6 (-4, 0) -> (-9.3, 6.5)
  line L7 (-9.3, 6.5) -> (-9.3, 0) projected
  line L8 (-4, 6.5) -> (-9.3, 0)
  point P0 (0, 6.5)
  point P1 (-6.65, 3.25)
  dimension "d217" = 5.3
  constraints: 6 end point, 2 midpoint, 2 point on line, 1 perpendicular
  measures "d217" distance between parallel lines of L2 L4
hole "Hole4" at (27.5, -3.25, 6.65) direction (-1, 0, 0) diameter 2.459 depth 10 thread size "M3x0.5" class "6H" standard "ISO Metric profile"
sketch "Sketch5" plane through (0, -66.431155, 0) normal (-1, 0, 0) x (0, 0, 1)
  line L0 (0, 40.288851) -> (0, 20.644607)
  line L1 (0, 40.288851) -> (-3.8, 40.288851)
  line L2 (0, 20.644607) -> (-3.8, 20.644607)
  line L3 (-3.8, 40.288851) -> (-3.8, 20.644607)
  circle A0 centre (-1.9, 30.966729) radius 1.0065
  point P0 (0, 66.431155)
hole "Hole3" [suppressed]
sketch "Sketch7" plane through (23.2, -66.431155, 9.3) normal (1, 0, 0) x (0, 0, -1)
  line L0 (9.3, 59.931155) -> (0, 59.931155)
  line L1 (0, 59.931155) -> (0, 0)
  line L2 (9.3, 0) -> (0, 0)
  circle A0 centre (6.55, 54.201655) radius 2.75
  line L3 (9.3, 59.931155) -> (0, 59.931155)
  circle A1 centre (6.55, 6.75) radius 2.75
  line L4 (5.3, 19.749714) -> (9.3, 19.749714)
  line L5 (9.3, 19.749714) -> (9.3, 59.931155)
  line L6 (9.3, 4) -> (9.3, 15.599965)
  line L7 (9.3, 1) -> (5.3, 1)
  line L8 (5.3, 4) -> (9.3, 4)
  line L9 (9.3, 0) -> (9.3, 1)
  line L10 (5.3, 15.599965) -> (5.3, 19.749714)
  line L11 (9.3, 58.160655) -> (9.3, 55.701655)
  line L12 (0, 55.701655) -> (0, 58.160655)
  line L13 (5.3, 1) -> (5.3, 4)
  line L14 (9.3, 15.599965) -> (5.3, 15.599965)
  point P0 (9.3, 66.431155)
  dimension "d122" = 5.5
  dimension "d123" = 5.5
  dimension "d194" = 1.5
  constraints: 3 tangent, 2 centre point
  measures "d122" diameter of A0
  measures "d123" diameter of A1
  measures "d194" vertical distance of A0.centre L11.end
hole "Hole5" at (23.2, -59.681155, 2.75) at (23.2, -12.2295, 2.75) direction (-1, 0, 0) diameter 2.013 depth 8 thread size "M2.5x0.45" class "6H" standard "ISO Metric profile"